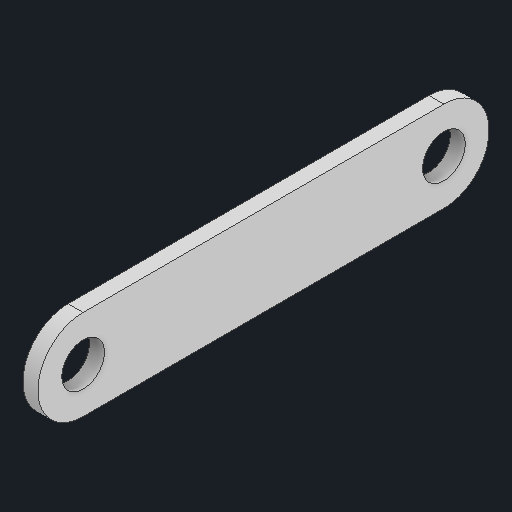
# Autodesk Inventor part: Motor Gearbox Gusset
Saved by Autodesk Inventor 2025 (Build 290162000, 162)
## iProperties
Created: 2024-12-31
Part Number: Motor Gearbox Gusset
Material: Generic
Document SubType Name: Modeling
Designer: Averey Ku
Density: 1 g/cm^3
Appearance: Default
Author: Averey Ku
Autodesk Inventor part; units mm, degrees
ref_plane "YZ Plane" through (0, 0, 0) normal (1, 0, 0) x (0, 1, 0)
ref_plane "XZ Plane" through (0, 0, 0) normal (0, 1, 0) x (-1, 0, 0)
ref_plane "XY Plane" through (0, 0, 0) normal (0, 0, 1) x (1, 0, 0)
sketch "Sketch1" plane through (0, 0, 0) normal (1, 0, 0) x (0, 1, 0)
  circle A0 centre (0, 0) radius 2.2479
  circle A1 centre (0, -38.1) radius 2.2479
  arc A2 (4.7625, 0) -> (-4.7625, 0) centre (0, 0) ccw
  arc A3 (-4.7625, -38.1) -> (4.7625, -38.1) centre (0, -38.1) ccw
  line L0 (4.7625, 0) -> (4.7625, -38.1)
  line L1 (-4.7625, -38.1) -> (-4.7625, 0)
  dimension "d0" = 4.4958
  dimension "d1" = 4.4958
  dimension "d2" = 9.525
  dimension "d3" = 9.525
  constraints: 4 centre point, 4 end point, 4 point on circle, 3 coincident, 1 parallel, 1 tangent
  measures "d0" diameter of A0
  measures "d1" diameter of A1
  measures "d2" diameter of A2
  measures "d3" diameter of A3
extrude "Extrusion1" add sketch "Sketch1" along normal blind 1.5875
body "Solid1"
